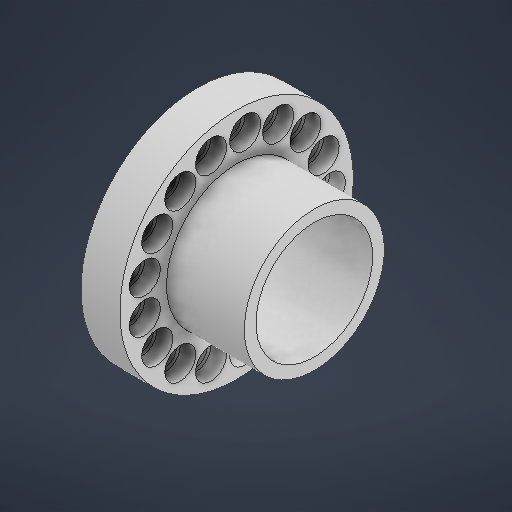
# Autodesk Inventor part: Part3
Saved by Autodesk Inventor 2026 (Build 300175050, 175E)
## iProperties
Created: 2026-04-16
Part Number: Part3
Material: Generic
Document SubType Name: Modeling
Designer: Administrator
Density: 1 g/cm^3
Appearance: Default
Author: Administrator
Autodesk Inventor part; units mm, degrees
ref_plane "YZ Plane" through (0, 0, 0) normal (1, 0, 0) x (0, 1, 0)
ref_plane "XZ Plane" through (0, 0, 0) normal (0, 1, 0) x (-1, 0, 0)
ref_plane "XY Plane" through (0, 0, 0) normal (0, 0, 1) x (1, 0, 0)
sketch "Sketch1" plane through (0, 0, 0) normal (1, 0, 0) x (0, 1, 0)
  circle A0 centre (0, 0) radius 15
  circle A1 centre (0, 0) radius 9
  circle A2 centre (0, 0) radius 7.5
  dimension "d0" = 15
  dimension "d1" = 18
  dimension "d2" = 30
  constraints: 3 centre point, 3 coincident
  measures "d0" diameter of A2
  measures "d1" diameter of A1
  measures "d2" diameter of A0
extrude "Extrusion1" add sketch "Sketch1" against normal blind 5 contours A0 | A1
extrude "Extrusion2" add sketch "Sketch1" along normal blind 10 contours A1
sketch "Sketch2" plane through (0, 0, 0) normal (1, 0, 0) x (0, 0, -1)
  point P0 (0, 0)
  point P1 (0, 0)
  point P2 (12, 0)
  dimension "d7" = 12
  constraints: 1 coincident
  measures "d7" distance of point (0, 0) point (12, 0)
hole "Hole1" at (0, 0, 0) at (0, 0, -12) direction (-1, 0, 0) diameter 3 end through all counterbore diameter 4 counterbore depth 2
pattern_circular "Circular Pattern1" count 17 over 360 about axis through (0, 0, 0) along (-1, 0, 0) of "Hole1"
body "Solid1"
